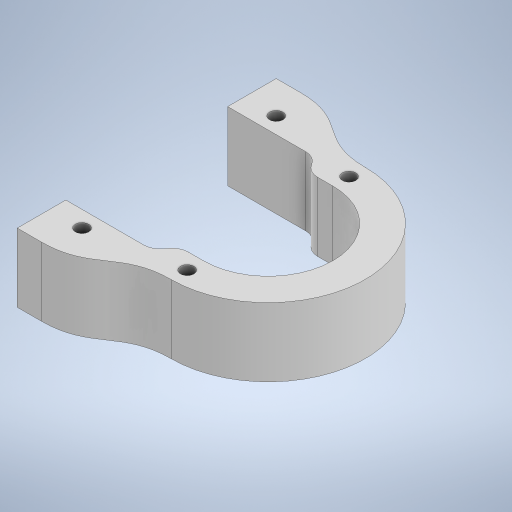
# Autodesk Inventor part: L1 Gearbox Cover
Saved by Autodesk Inventor 2024 (Build 280153000, 153)
## iProperties
Created: 2023-09-26
Part Number: L1 Gearbox Cover
Material: Generic
Document SubType Name: Modeling
Designer: lando
Density: 1 g/cm^3
Appearance: Default
Author: lando
Autodesk Inventor part; units mm, degrees
ref_plane "YZ Plane" through (0, 0, 0) normal (1, 0, 0) x (0, 1, 0)
ref_plane "XZ Plane" through (0, 0, 0) normal (0, 1, 0) x (-1, 0, 0)
ref_plane "XY Plane" through (0, 0, 0) normal (0, 0, 1) x (1, 0, 0)
sketch "Sketch1" plane through (0, 0, 0) normal (0, 1, 0) x (-1, 0, 0)
  line L0 (99.4671, -212.1342) -> (-395.7488, 283.0816) construction
  circle A0 centre (-24.2079, -174.0342) radius 2.65
  circle A1 centre (-21.0329, -212.1342) radius 6.35
  circle A2 centre (1.1921, -174.0342) radius 2.65
  circle A3 centre (10.7171, -212.1342) radius 14.2875
  circle A4 centre (26.5921, -174.0342) radius 2.65
  line L1 (-84.5329, -212.1342) -> (10.7171, -212.1342) construction
  line L2 (39.2921, -161.3342) -> (-113.1079, -161.3342)
  line L3 (-113.1079, -262.9342) -> (39.2921, -262.9342)
  circle A5 centre (-49.6079, -174.0342) radius 2.65
  circle A6 centre (-52.7829, -212.1342) radius 6.35
  circle A7 centre (-75.0079, -174.0342) radius 2.65
  circle A8 centre (-75.0079, -250.2342) radius 2.65
  circle A9 centre (-84.5329, -212.1342) radius 14.2875
  circle A10 centre (-100.4079, -174.0342) radius 2.65
  circle A11 centre (-100.4079, -250.2342) radius 2.65
  circle A12 centre (-49.6079, -250.2342) radius 2.65
  circle A13 centre (1.1921, -250.2342) radius 2.65
  circle A14 centre (26.5921, -250.2342) radius 2.65
  circle A15 centre (-24.2079, -250.2342) radius 2.65
  line L4 (39.2921, -262.9342) -> (39.2921, -161.3342)
  line L5 (39.2921, -237.5342) -> (395.5271, -237.5342)
  line L6 (74.0671, -186.7342) -> (39.2921, -186.7342)
  line L7 (-113.1079, -161.3342) -> (-113.1079, -262.9342)
  spline S0 degree 3 poles (-84.5329, -174.0342) (-65.4829, -174.0342) (-65.4829, -161.3342) (-46.4329, -161.3342) knots 1 1 1 1 2 2 2 2
  line L8 (-84.5329, -174.0342) -> (-65.4829, -174.0342) construction
  line L9 (-65.4829, -174.0342) -> (-65.4829, -161.3342) construction
  line L10 (-65.4829, -161.3342) -> (-46.4329, -161.3342) construction
  circle A16 centre (-84.5329, -212.1342) radius 38.1
  circle A17 centre (-84.5329, -180.3842) radius 2.65
  spline S1 degree 3 poles (-84.5329, -250.2342) (-65.4829, -250.2342) (-65.4829, -262.9342) (-46.4329, -262.9342) knots 1 1 1 1 2 2 2 2
  line L11 (-84.5329, -250.2342) -> (-65.4829, -250.2342) construction
  line L12 (-65.4829, -250.2342) -> (-65.4829, -262.9342) construction
  line L13 (-65.4829, -262.9342) -> (-46.4329, -262.9342) construction
  circle A18 centre (-84.5329, -243.8842) radius 2.65
  point P0 (0, 0)
  point P1 (-36.9079, -262.9342)
  point P2 (-36.9079, -212.1342)
  point P3 (39.2921, -212.1342)
  point P4 (-46.4329, -262.9342)
  point P5 (-46.4329, -161.3342)
  dimension "d0" = 31.75
  constraints: 18 centre point, 16 end point, 4 point on line, 1 equal radius, 1 vertical alignment, 9 other
  measures "d0" distance of A18.centre L1.start
extrude "Extrusion1" add sketch "Sketch1" along normal blind 26.924 contours L4 L3 S1 A8 A16 A7 S0 L2 | A7 A16 S0 | A16 A7 A8 L7 | L7 A16 | A7 A16 S0 | A7 A16 | A16 A8 S1 | S1 A8 A16 | A8 A16
sketch "Sketch2" plane through (0, 26.924, 0) normal (0, 1, 0) x (1, 0, 0)
  circle A0 centre (49.6079, 174.0342) radius 2.65 projected
  circle A1 centre (49.6079, 174.0342) radius 2.65
  line L0 (49.6079, 174.0342) -> (36.9079, 174.0342)
  line L1 (-39.2921, 161.3342) -> (46.4329, 161.3342) projected
  line L2 (36.9079, 161.3342) -> (36.9079, 271.4653)
  line L3 (36.9079, 271.4653) -> (-75.2217, 284.061)
  line L4 (-75.2217, 284.061) -> (-39.9967, 13.0358)
  line L5 (-39.9967, 13.0358) -> (36.9079, 161.3342)
  point P0 (0, 0)
  dimension "d3" = 12.7
  constraints: 10 end point, 1 centre point, 1 coincident, 1 horizontal, 1 point on line, 1 vertical
  measures "d3" distance of L0.start L0.end
extrude "Extrusion2" cut sketch "Sketch2" against normal blind 26.924 contours L5 L4 L3 L2
sketch "Sketch3" plane through (0, 26.924, 0) normal (0, 1, 0) x (1, 0, 0)
  line L0 (26.0555, 454.6039) -> (26.0555, 378.7664)
  line L1 (26.0555, 454.6039) -> (26.0555, 378.7664)
  arc A0 (38.7555, 340.6664) -> (114.9555, 340.6664) centre (76.8555, 340.6664) ccw
  circle A1 centre (76.8555, 340.6664) radius 38.1
  line L2 (26.0555, 378.7664) -> (45.1055, 378.7664)
  line L3 (45.1055, 357.6525) -> (45.1055, 454.6039)
  arc A2 (51.4555, 340.6664) -> (102.2555, 340.6664) centre (76.8555, 340.6664) ccw
  line L4 (45.1055, 378.7664) -> (51.4555, 378.7664)
  line L5 (51.4555, 346.6539) -> (51.4555, 340.6664)
  line L6 (45.1055, 353.0039) -> (45.1055, 353.0039)
  arc A3 (51.4555, 346.6539) -> (48.2805, 352.1532) centre (45.1055, 346.6539) ccw
  arc A4 (45.1055, 357.6525) -> (48.2805, 352.1532) centre (51.4555, 357.6525) ccw
  line L7 (108.6055, 357.6525) -> (108.6055, 454.6039)
  arc A5 (105.4305, 352.1532) -> (102.2555, 346.6539) centre (108.6055, 346.6539) ccw
  arc A6 (105.4305, 352.1532) -> (108.6055, 357.6525) centre (102.2555, 357.6525) ccw
  line L8 (102.2555, 346.6539) -> (102.2555, 340.6664)
  line L9 (127.6555, 378.7664) -> (127.6555, 454.8164)
  line L10 (127.6555, 454.8164) -> (127.6555, 337.8192)
  spline S0 degree 3 poles (26.0555, 378.7664) (26.0555, 359.7164) (38.7555, 359.7164) (38.7555, 340.6664) knots 1 1 1 1 2 2 2 2
  line L11 (26.0555, 378.7664) -> (26.0555, 359.7164) construction
  line L12 (26.0555, 359.7164) -> (38.7555, 359.7164) construction
  line L13 (38.7555, 359.7164) -> (38.7555, 340.6664) construction
  line L14 (76.8555, 340.6664) -> (76.8555, 373.056)
  spline S1 degree 3 poles (127.6555, 378.7664) (127.6555, 359.7164) (114.9555, 359.7164) (114.9555, 340.6664) knots 1 1 1 1 2 2 2 2
  line L15 (127.6555, 378.7664) -> (127.6555, 359.7164) construction
  line L16 (127.6555, 359.7164) -> (114.9555, 359.7164) construction
  line L17 (114.9555, 359.7164) -> (114.9555, 340.6664) construction
  circle A7 centre (38.7555, 400.9914) radius 2.65
  circle A8 centre (38.7555, 400.9914) radius 2.65
  circle A9 centre (38.7555, 375.5914) radius 2.65
  circle A10 centre (38.7555, 375.5914) radius 2.65
  circle A11 centre (45.1055, 340.6664) radius 2.65
  circle A12 centre (45.1055, 340.6664) radius 2.65
  circle A13 centre (108.6055, 340.6664) radius 2.65
  circle A14 centre (108.6055, 340.6664) radius 2.65
  circle A15 centre (114.9555, 375.5914) radius 2.65
  circle A16 centre (114.9555, 375.5914) radius 2.65
  circle A17 centre (114.9555, 400.9914) radius 2.65
  circle A18 centre (114.9555, 400.9914) radius 2.65
  circle A19 centre (76.8555, 308.9164) radius 2.65
  circle A20 centre (76.8555, 308.9164) radius 2.65
  line L18 (70.868, 315.2664) -> (76.8555, 315.2664)
  arc A21 (70.868, 315.2664) -> (65.3687, 312.0914) centre (70.868, 308.9164) ccw
  line L19 (64.518, 308.9164) -> (64.518, 308.9164)
  arc A22 (59.8694, 308.9164) -> (65.3687, 312.0914) centre (59.8694, 315.2664) ccw
  line L20 (57.8055, 302.5664) -> (76.8555, 302.5664) construction
  spline S2 degree 3 poles (38.7555, 289.8664) (57.8055, 289.8664) (57.8055, 302.5664) (76.8555, 302.5664) knots 1 1 1 1 2 2 2 2
  line L21 (38.7555, 289.8664) -> (57.8055, 289.8664) construction
  line L22 (57.8055, 289.8664) -> (57.8055, 302.5664) construction
  line L23 (38.7555, 308.9164) -> (38.7555, 315.2664)
  line L24 (38.7555, 289.8664) -> (38.7555, 308.9164)
  circle A23 centre (41.9305, 302.5664) radius 2.65
  line L25 (-37.082, 289.8664) -> (38.7555, 289.8664)
  line L26 (-37.082, 289.8664) -> (38.7555, 289.8664)
  line L27 (59.8694, 308.9164) -> (-37.082, 308.9164)
  line L28 (59.8694, 372.4164) -> (-37.082, 372.4164)
  circle A24 centre (16.5305, 378.7664) radius 2.65
  circle A25 centre (16.5305, 378.7664) radius 2.65
  line L29 (-37.2945, 391.4664) -> (79.7027, 391.4664)
  line L30 (38.7555, 391.4664) -> (-37.2945, 391.4664)
  circle A26 centre (16.5305, 302.5664) radius 2.65
  circle A27 centre (16.5305, 302.5664) radius 2.65
  circle A28 centre (41.9305, 302.5664) radius 2.65
  circle A29 centre (41.9305, 378.7664) radius 2.65
  circle A30 centre (41.9305, 378.7664) radius 2.65
  line L31 (38.7555, 391.4664) -> (57.8055, 391.4664) construction
  spline S3 degree 3 poles (38.7555, 391.4664) (57.8055, 391.4664) (57.8055, 378.7664) (76.8555, 378.7664) knots 1 1 1 1 2 2 2 2
  line L32 (57.8055, 391.4664) -> (57.8055, 378.7664) construction
  line L33 (57.8055, 378.7664) -> (76.8555, 378.7664) construction
  arc A31 (65.3687, 369.2414) -> (59.8694, 372.4164) centre (59.8694, 366.0664) ccw
  arc A32 (65.3687, 369.2414) -> (70.868, 366.0664) centre (70.868, 372.4164) ccw
  line L34 (70.868, 366.0664) -> (76.8555, 366.0664)
  circle A33 centre (76.8555, 372.4164) radius 2.65
  circle A34 centre (76.8555, 372.4164) radius 2.65
  arc A35 (76.8555, 302.5664) -> (76.8555, 378.7664) centre (76.8555, 340.6664) ccw
  circle A36 centre (76.8555, 340.6664) radius 38.1
  line L35 (76.8555, 340.6664) -> (44.4659, 340.6664)
  arc A37 (76.8555, 315.2664) -> (76.8555, 366.0664) centre (76.8555, 340.6664) ccw
  circle A38 centre (84.5329, 212.1342) radius 14.2875 projected
  circle A39 centre (84.5329, 212.1342) radius 14.2875
  circle A40 centre (52.7829, 212.1342) radius 2.65
  circle A41 centre (52.7829, 212.1342) radius 2.65
  line L36 (59.1329, 218.1218) -> (59.1329, 212.1342)
  arc A42 (59.1329, 218.1218) -> (55.9579, 223.6211) centre (52.7829, 218.1218) ccw
  line L37 (52.7829, 224.4718) -> (52.7829, 224.4718)
  arc A43 (52.7829, 229.1203) -> (55.9579, 223.6211) centre (59.1329, 229.1203) ccw
  line L38 (46.4329, 231.1842) -> (46.4329, 212.1342) construction
  spline S4 degree 3 poles (33.7329, 250.2342) (33.7329, 231.1842) (46.4329, 231.1842) (46.4329, 212.1342) knots 1 1 1 1 2 2 2 2
  line L39 (33.7329, 250.2342) -> (33.7329, 231.1842) construction
  line L40 (33.7329, 231.1842) -> (46.4329, 231.1842) construction
  line L41 (52.7829, 250.2342) -> (59.1329, 250.2342)
  line L42 (33.7329, 250.2342) -> (52.7829, 250.2342)
  circle A44 centre (46.4329, 247.0592) radius 2.65
  line L43 (33.7329, 326.0718) -> (33.7329, 250.2342)
  line L44 (33.7329, 326.0718) -> (33.7329, 250.2342)
  line L45 (52.7829, 229.1203) -> (52.7829, 326.0718)
  line L46 (116.2829, 229.1203) -> (116.2829, 326.0718)
  circle A45 centre (122.6329, 272.4592) radius 2.65
  circle A46 centre (122.6329, 272.4592) radius 2.65
  line L47 (135.3329, 326.2842) -> (135.3329, 209.2871)
  line L48 (135.3329, 250.2342) -> (135.3329, 326.2842)
  circle A47 centre (46.4329, 272.4592) radius 2.65
  circle A48 centre (46.4329, 272.4592) radius 2.65
  circle A49 centre (46.4329, 247.0592) radius 2.65
  circle A50 centre (122.6329, 247.0592) radius 2.65
  circle A51 centre (122.6329, 247.0592) radius 2.65
  line L49 (135.3329, 250.2342) -> (135.3329, 231.1842) construction
  spline S5 degree 3 poles (135.3329, 250.2342) (135.3329, 231.1842) (122.6329, 231.1842) (122.6329, 212.1342) knots 1 1 1 1 2 2 2 2
  line L50 (135.3329, 231.1842) -> (122.6329, 231.1842) construction
  line L51 (122.6329, 231.1842) -> (122.6329, 212.1342) construction
  arc A52 (113.1079, 223.6211) -> (116.2829, 229.1203) centre (109.9329, 229.1203) ccw
  arc A53 (113.1079, 223.6211) -> (109.9329, 218.1218) centre (116.2829, 218.1218) ccw
  line L52 (109.9329, 218.1218) -> (109.9329, 212.1342)
  circle A54 centre (116.2829, 212.1342) radius 2.65
  circle A55 centre (116.2829, 212.1342) radius 2.65
  arc A56 (46.4329, 212.1342) -> (122.6329, 212.1342) centre (84.5329, 212.1342) ccw
  circle A57 centre (84.5329, 212.1342) radius 38.1
  line L53 (84.5329, 212.1342) -> (84.5329, 244.5238)
  arc A58 (59.1329, 212.1342) -> (109.9329, 212.1342) centre (84.5329, 212.1342) ccw
  line L54 (78.5454, 237.5342) -> (84.5329, 237.5342)
  arc A59 (73.0461, 240.7092) -> (78.5454, 237.5342) centre (78.5454, 243.8842) ccw
  line L55 (84.5329, 212.1342) -> (52.1434, 212.1342)
  arc A60 (84.5329, 186.7342) -> (84.5329, 237.5342) centre (84.5329, 212.1342) ccw
  circle A61 centre (84.5329, 212.1342) radius 38.1
  arc A62 (84.5329, 174.0342) -> (84.5329, 250.2342) centre (84.5329, 212.1342) ccw
  line L56 (78.5454, 186.7342) -> (84.5329, 186.7342)
  arc A63 (78.5454, 186.7342) -> (73.0461, 183.5592) centre (78.5454, 180.3842) ccw
  line L57 (72.1954, 180.3842) -> (72.1954, 180.3842)
  arc A64 (67.5469, 180.3842) -> (73.0461, 183.5592) centre (67.5469, 186.7342) ccw
  circle A65 centre (84.5329, 180.3842) radius 2.65
  circle A66 centre (84.5329, 180.3842) radius 2.65
  line L58 (65.4829, 174.0342) -> (84.5329, 174.0342) construction
  spline S6 degree 3 poles (46.4329, 161.3342) (65.4829, 161.3342) (65.4829, 174.0342) (84.5329, 174.0342) knots 1 1 1 1 2 2 2 2
  line L59 (46.4329, 161.3342) -> (65.4829, 161.3342) construction
  line L60 (65.4829, 161.3342) -> (65.4829, 174.0342) construction
  line L61 (46.4329, 180.3842) -> (46.4329, 186.7342)
  circle A67 centre (84.5329, 243.8842) radius 2.65
  circle A68 centre (84.5329, 243.8842) radius 2.65
  line L62 (65.4829, 250.2342) -> (84.5329, 250.2342) construction
  spline S7 degree 3 poles (46.4329, 262.9342) (65.4829, 262.9342) (65.4829, 250.2342) (84.5329, 250.2342) knots 1 1 1 1 2 2 2 2
  line L63 (46.4329, 262.9342) -> (65.4829, 262.9342) construction
  line L64 (65.4829, 262.9342) -> (65.4829, 250.2342) construction
  circle A69 centre (49.6079, 250.2342) radius 2.65
  circle A70 centre (49.6079, 250.2342) radius 2.65
  arc A71 (73.0461, 240.7092) -> (67.5469, 243.8842) centre (67.5469, 237.5342) ccw
  line L65 (46.4329, 161.3342) -> (46.4329, 180.3842)
  circle A72 centre (49.6079, 174.0342) radius 2.65
  line L66 (-29.4046, 161.3342) -> (46.4329, 161.3342)
  line L67 (-29.4046, 161.3342) -> (46.4329, 161.3342)
  line L68 (67.5469, 180.3842) -> (-29.4046, 180.3842)
  line L69 (67.5469, 243.8842) -> (-29.4046, 243.8842)
  circle A73 centre (24.2079, 250.2342) radius 2.65
  circle A74 centre (24.2079, 250.2342) radius 2.65
  line L70 (-29.6171, 262.9342) -> (87.3801, 262.9342)
  line L71 (46.4329, 262.9342) -> (-29.6171, 262.9342)
  circle A75 centre (49.6079, 174.0342) radius 2.65
  circle A76 centre (24.2079, 174.0342) radius 2.65
  circle A77 centre (24.2079, 174.0342) radius 2.65
  line L72 (-29.4046, 180.3842) -> (-29.4046, 243.8842)
  point P0 (0, 0)
  point P1 (161.6667, 205.692)
  point P2 (36.9079, 161.3342)
  point P3 (71.58, 306.9082)
  point P4 (46.4329, 161.3342)
  point P5 (110.6137, 335.3909)
  point P6 (79.2575, 178.376)
  point P7 (118.2912, 206.8588)
  dimension "d9" = 19.05
  dimension "d10" = 12.7
  dimension "d11" = 76.2
  dimension "d12" = 101.6
  dimension "d13" = 6.35
  dimension "d14" = 19.05
  dimension "d15" = 19.05
  dimension "d16" = 19.05
  dimension "d17" = 12.7
  dimension "d18" = 76.2
  dimension "d19" = 101.6
  dimension "d20" = 6.35
  dimension "d21" = 19.05
  dimension "d22" = 19.05
  dimension "d23" = 19.05
  dimension "d24" = 12.7
  dimension "d25" = 76.2
  dimension "d26" = 101.6
  dimension "d27" = 6.35
  dimension "d28" = 19.05
  dimension "d29" = 19.05
  dimension "d30" = 19.05
  dimension "d31" = 12.7
  dimension "d32" = 76.2
  dimension "d33" = 101.6
  dimension "d34" = 6.35
  dimension "d35" = 19.05
  dimension "d36" = 19.05
  constraints: 98 end point, 77 centre point, 52 point on circle, 29 coincident, 20 tangent, 16 symmetric about line, 12 perpendicular, 9 vertical, 8 point on line, 4 concentric, 4 equal radius, 4 horizontal, 4 parallel, 24 other
  measures "d9" distance of L2.end L2.start
  measures "d10" radial gap between concentric circles of A0 A2
  measures "d11" diameter of A1
  measures "d12" distance of L6.start L3.end
  measures "d13" radius of A3
  measures "d14" distance of L11.start L11.end
  measures "d15" distance of L13.end L13.start
  measures "d16" distance of L24.end L24.start
  measures "d17" radial gap between concentric circles of A35 A37
  measures "d18" diameter of A36
  measures "d19" distance of L19.start L27.end
  measures "d20" radius of A21
  measures "d21" distance of L21.start L21.end
  measures "d22" distance of L20.end L20.start
  measures "d23" distance of L42.end L43.end
  measures "d24" radial gap between concentric circles of A56 A58
  measures "d25" diameter of A57
  measures "d26" distance of L37.start L45.end
  measures "d27" radius of A42
  measures "d28" distance of L39.start L39.end
  measures "d29" distance of L38.end L38.start
  measures "d30" distance of L65.end L66.end
  measures "d31" radial gap between concentric circles of A62 A60
  measures "d32" diameter of A61
  measures "d33" distance of L57.start L68.end
  measures "d34" radius of A63
  measures "d35" distance of L59.start L59.end
  measures "d36" distance of L58.end L60.end
extrude "Extrusion3" cut sketch "Sketch3" against normal blind 26.924 contours L69 A57 L45 | L45 A57 S4 L69 | L69 A71 A59 L54 L53 A38 L55 L36 A42 A43 L45 A57 | S4 A56 L68 L72 L69 | L45 A43 A42 L36 A58 L56 A63 A64 L68 A56 A57 | A58 L55 A38 L53 A60
body "Solid1"
